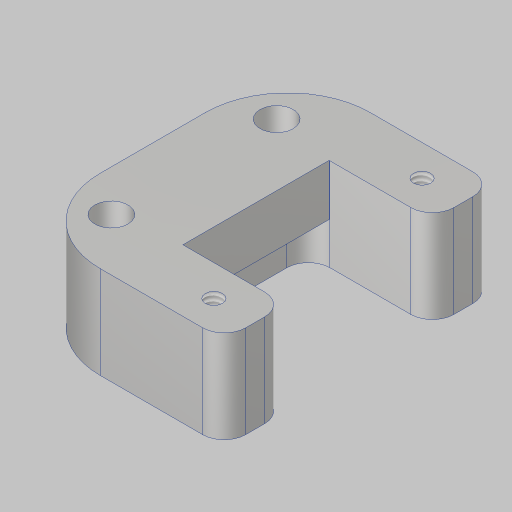
# Autodesk Inventor part: GP7-006
Saved by Autodesk Inventor 2023.5 (Build 275446000, 446)
## iProperties
Created: 2025-02-25
Part Number: GP7-006
Material: Aluminum 6061
Document SubType Name: Modeling
Designer: slick
Density: 2.7 g/cm^3
Appearance: Aluminum - Flat
Author: slick
Autodesk Inventor part; units mm, degrees
ref_plane "YZ Plane" through (0, 0, 0) normal (1, 0, 0) x (0, 1, 0)
ref_plane "XZ Plane" through (0, 0, 0) normal (0, 1, 0) x (-1, 0, 0)
ref_plane "XY Plane" through (0, 0, 0) normal (0, 0, 1) x (1, 0, 0)
sketch "Sketch1" plane through (0, 0, 0) normal (1, 0, 0) x (0, 1, 0)
  line L0 (0, 20.7625) -> (0, -20.7625)
  line L1 (0, 20.7625) -> (14.224, 20.7625)
  line L2 (14.224, 20.7625) -> (14.224, 11.2375)
  line L3 (14.224, 11.2375) -> (6.35, 11.2375)
  line L4 (6.35, 11.2375) -> (6.35, -11.2375)
  line L5 (6.35, -11.2375) -> (14.224, -11.2375)
  line L6 (14.224, -11.2375) -> (14.224, -20.7625)
  line L7 (14.224, -20.7625) -> (0, -20.7625)
  point P0 (0, 0)
  point P1 (0, 0)
  point P2 (14.224, -16)
  point P3 (14.224, 16)
  dimension "d1" = 32
  dimension "d2" = 7.874
  dimension "d4" = 6.35
  dimension "d5" = 9.525
  constraints: 16 end point, 6 perpendicular, 3 midpoint, 2 coincident, 1 collinear, 1 horizontal, 1 vertical, 1 vertical alignment
  measures "d1" distance of point (14.224, -16) point (14.224, 16)
  measures "d2" distance of L2.end L3.end
  measures "d4" distance between parallel lines of L0 L4
  measures "d5" distance between parallel lines of L3 L1
extrude "Extrusion1" add sketch "Sketch1" along normal blind 31.75
sketch "Sketch2" plane through (0, 14.224, 20.7625) normal (0, 1, 0) x (1, 0, 0)
  line L0 (0, 9.525) -> (31.75, 9.525) construction
  line L1 (31.75, 9.525) -> (31.75, 0) construction
  line L2 (31.75, 0) -> (0, 0) construction
  line L3 (0, 0) -> (0, 9.525) construction
  line L4 (0, 41.525) -> (31.75, 41.525) construction
  line L5 (31.75, 41.525) -> (31.75, 32) construction
  line L6 (31.75, 32) -> (0, 32) construction
  line L7 (0, 32) -> (0, 41.525) construction
  point P0 (0, 20.7625)
  point P1 (25.4, 4.7625)
  point P2 (25.4, 36.7625)
  point P3 (31.75, 4.7625)
  point P4 (31.75, 36.7625)
  dimension "d8" = 6.35
  constraints: 2 horizontal alignment, 2 midpoint, 1 vertical alignment
  measures "d8" distance from line of L1 point (25.4, 4.762)
hole "Hole1" at (25.4, 14.224, 16) at (25.4, 14.224, -16) direction (0, -1, 0) diameter 2.6416 end through all thread size "6-32 UNC" class "2B" standard "ANSI Unified Screw Threads"
sketch "Sketch4" plane through (0, 6.35, 11.2375) normal (0, 1, 0) x (1, 0, 0)
  circle A0 centre (25.4, -4.7625) radius 1.3208 construction
  circle A1 centre (25.4, 27.2375) radius 1.3208 construction
  line L0 (0, 32) -> (31.75, 32) construction
  line L1 (31.75, 32) -> (31.75, 22.475) construction
  line L2 (31.75, 22.475) -> (0, 22.475) construction
  line L3 (0, 0) -> (0, 22.475) construction
  line L4 (0, 0) -> (31.75, 0) construction
  line L5 (31.75, 0) -> (31.75, -9.525) construction
  line L6 (31.75, -9.525) -> (0, -9.525) construction
  line L7 (0, -9.525) -> (0, 0) construction
  line L8 (0, 22.475) -> (0, 32) construction
  line L9 (31.75, 22.475) -> (31.75, 0) construction
  line L10 (0, 22.475) -> (31.75, 22.475) construction
  line L11 (31.75, 0) -> (12.7, 0)
  line L12 (12.7, 0) -> (12.7, 22.475)
  line L13 (12.7, 22.475) -> (31.75, 22.475)
  line L14 (31.75, 22.475) -> (31.75, 0)
  point P0 (0, 11.2375)
  point P1 (14.7922, 22.475)
  dimension "d25" = 19.05
  constraints: 8 end point, 2 parallel, 1 horizontal, 1 perpendicular, 1 point on line
  measures "d25" distance between parallel lines of L9 L12
extrude "Extrusion2" cut sketch "Sketch4" against normal blind 38.1
sketch "Sketch5" plane through (0, 14.224, 20.7625) normal (0, 1, 0) x (1, 0, 0)
  line L0 (0, 0) -> (0, 41.525) construction
  line L1 (0, 41.525) -> (31.75, 41.525) construction
  line L2 (0, 0) -> (15.875, 0)
  line L3 (15.875, 0) -> (15.875, 41.525)
  line L4 (15.875, 41.525) -> (0, 41.525)
  line L5 (0, 41.525) -> (0, 0)
  point P0 (0, 20.7625)
  constraints: 8 end point, 2 parallel, 1 horizontal, 1 midpoint, 1 perpendicular
extrude "Extrusion3" add sketch "Sketch5" against normal up to surface (7.874 mm away)
sketch "Sketch6" plane through (0, 14.224, 20.7625) normal (0, 1, 0) x (1, 0, 0)
  line L0 (6.35, 8.0625) -> (6.35, 33.4625) construction
  line L1 (0, 41.525) -> (0, 0) construction
  point P0 (0, 20.7625)
  point P1 (6.35, 20.7625)
  point P2 (0, 20.7625)
  dimension "d30" = 6.35
  dimension "d31" = 25.4
  constraints: 2 end point, 2 midpoint, 1 horizontal alignment, 1 vertical, 1 vertical alignment
  measures "d30" distance between parallel lines of L1 L0
  measures "d31" distance of L0.start L0.end
hole "Hole3" at (6.35, 14.224, 12.7) at (6.35, 14.224, -12.7) direction (0, -1, 0) diameter 5.1054 end through all clearance for "Flat Head Machine Screw (82)" size "#10" standard "Ansi Unified Screw Threads"
fillet "Fillet1" radius 12.7 2 edges at (0, 7.112, -20.7625) (0, 7.112, 20.7625)
fillet "Fillet2" radius 3.302 6 edges at (12.7, 3.175, -11.2375) (12.7, 3.175, 11.2375) (31.75, 7.112, 20.7625) (31.75, 7.112, 11.2375) (31.75, 7.112, -11.2375) (31.75, 7.112, -20.7625)
body "Solid1"
